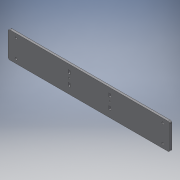
# Autodesk Inventor part: Motor Brace_1
Saved by Autodesk Inventor 2019 (Build 230136000, 136)
## iProperties
Created: 2020-03-11
Part Number: Motor Brace_1
Material: Generic
Document SubType Name: Modeling
Designer: Vijay
Density: 1 g/cm^3
Appearance: Default
Author: Vijay
Autodesk Inventor part; units mm, degrees
ref_plane "YZ Plane" through (0, 0, 0) normal (1, 0, 0) x (0, 1, 0)
ref_plane "XZ Plane" through (0, 0, 0) normal (0, 1, 0) x (-1, 0, 0)
ref_plane "XY Plane" through (0, 0, 0) normal (0, 0, 1) x (1, 0, 0)
sketch "Sketch1" plane through (0, 0, 0) normal (0, 0, 1) x (1, 0, 0)
  line L0 (-283, 0) -> (-283, -900) projected
  line L1 (26, 100) -> (26, -900) projected
  line L2 (-283, -450) -> (26, -450)
  line L3 (26, -450) -> (26, -400)
  line L4 (26, -400) -> (-283, -400)
  line L5 (-283, -400) -> (-283, -450)
  point P0 (0, 0)
  dimension "d0" = 50
  constraints: 8 end point, 2 midpoint, 2 parallel, 1 horizontal, 1 perpendicular
  measures "d0" distance between parallel lines of L2 L4
extrude "Extrusion1" add sketch "Sketch1" along normal blind 4
fillet "Fillet1" radius 3.175 4 edges at (-283, -450, 2) (-283, -400, 2) (26, -450, 2) (26, -400, 2)
sketch "Sketch2" plane through (0, 0, 4) normal (0, 0, 1) x (1, 0, 0)
  line L0 (-90.6012, -437.2508) -> (-90.6012, -431.2508) construction
  line L1 (-90.6012, -437.2508) -> (-86.6012, -437.2508) construction
  line L2 (-86.6012, -431.2508) -> (-86.6012, -437.2508) construction
  line L3 (-90.6012, -431.2508) -> (-86.6012, -431.2508) construction
  line L4 (-90.6012, -416.0508) -> (-90.6012, -410.0508) construction
  line L5 (-90.6012, -416.0508) -> (-86.6012, -416.0508) construction
  line L6 (-86.6012, -410.0508) -> (-86.6012, -416.0508) construction
  line L7 (-90.6012, -410.0508) -> (-86.6012, -410.0508) construction
  line L8 (-168.3754, -437.2508) -> (-168.3754, -431.2508) construction
  line L9 (-168.3754, -437.2508) -> (-164.3754, -437.2508) construction
  line L10 (-164.3754, -431.2508) -> (-164.3754, -437.2508) construction
  line L11 (-168.3754, -431.2508) -> (-164.3754, -431.2508) construction
  line L12 (-168.3754, -416.0508) -> (-168.3754, -410.0508) construction
  line L13 (-168.3754, -416.0508) -> (-164.3754, -416.0508) construction
  line L14 (-164.3754, -410.0508) -> (-164.3754, -416.0508) construction
  line L15 (-168.3754, -410.0508) -> (-164.3754, -410.0508) construction
  line L16 (-112.9543, -436.0142) -> (-107.1133, -436.0142) construction
  line L17 (-168.3754, -425.1508) -> (-168.3754, -422.1508) construction
  line L18 (-168.3754, -425.1508) -> (-168.3754, -422.1508) construction
  line L19 (-168.3754, -425.1508) -> (-164.3754, -425.1508) construction
  line L20 (-164.3754, -422.1508) -> (-164.3754, -425.1508) construction
  line L21 (-168.3754, -422.1508) -> (-164.3754, -422.1508) construction
  line L22 (-90.6012, -425.1508) -> (-90.6012, -422.1508) construction
  line L23 (-90.6012, -425.1508) -> (-86.6012, -425.1508) construction
  line L24 (-86.6012, -422.1508) -> (-86.6012, -425.1508) construction
  line L25 (-90.6012, -422.1508) -> (-86.6012, -422.1508) construction
  line L26 (-86.5012, -431.1508) -> (-86.5012, -437.3508)
  line L27 (-86.5012, -437.3508) -> (-90.7012, -437.3508)
  line L28 (-90.7012, -437.3508) -> (-90.7012, -431.1508)
  line L29 (-90.7012, -431.1508) -> (-86.5012, -431.1508)
  line L30 (-86.5012, -416.1508) -> (-90.7012, -416.1508)
  line L31 (-90.7012, -416.1508) -> (-90.7012, -409.9508)
  line L32 (-90.7012, -409.9508) -> (-86.5012, -409.9508)
  line L33 (-86.5012, -409.9508) -> (-86.5012, -416.1508)
  line L34 (-164.2754, -437.3508) -> (-168.4754, -437.3508)
  line L35 (-168.4754, -437.3508) -> (-168.4754, -431.1508)
  line L36 (-168.4754, -431.1508) -> (-164.2754, -431.1508)
  line L37 (-164.2754, -431.1508) -> (-164.2754, -437.3508)
  line L38 (-164.2754, -416.1508) -> (-168.4754, -416.1508)
  line L39 (-168.4754, -416.1508) -> (-168.4754, -409.9508)
  line L40 (-168.4754, -409.9508) -> (-164.2754, -409.9508)
  line L41 (-164.2754, -409.9508) -> (-164.2754, -416.1508)
  circle A0 centre (-166.3754, -423.6508) radius 1.5
  circle A1 centre (-88.6012, -423.6508) radius 1.5
  point P0 (0, 0)
  dimension "d4" = 0.1
  dimension "d5" = 0.1
  dimension "d6" = 0.1
  dimension "d7" = 0.1
  dimension "d8" = 3
  dimension "d9" = 3
  constraints: 32 end point, 2 centre point, 12 other
  measures "d4" distance between parallel lines of L3 L29
  measures "d5" distance between parallel lines of L5 L30
  measures "d6" distance between parallel lines of L9 L34
  measures "d7" distance between parallel lines of L13 L38
  measures "d8" diameter of A0
  measures "d9" diameter of A1
extrude "Extrusion2" cut sketch "Sketch2" against normal through all
sketch "Sketch3" plane through (0, 0, 4) normal (0, 0, 1) x (1, 0, 0)
  line L0 (17.1, 100) -> (17.1, -900) projected
  line L1 (8.9, 100) -> (17.1, 100) projected
  line L2 (8.9, 100) -> (8.9, -900) projected
  line L3 (17.1, -900) -> (8.9, -900) projected
  line L4 (-263.9, 100) -> (-263.9, -900) projected
  line L5 (-272.1, 100) -> (-263.9, 100) projected
  line L6 (-272.1, 100) -> (-272.1, -900) projected
  line L7 (-263.9, -900) -> (-272.1, -900) projected
  line L8 (55.4545, -442) -> (-299.148, -442) construction
  line L9 (72.1451, -408) -> (-299.148, -408) construction
  line L10 (-279.825, -450) -> (22.825, -450) construction
  line L11 (22.825, -400) -> (-279.825, -400) construction
  line L12 (13, -462.5908) -> (13, -387.796) construction
  line L13 (-268, -463.1777) -> (-268, -383.364) construction
  circle A0 centre (13, -442) radius 2
  circle A1 centre (13, -408) radius 2
  circle A2 centre (-268, -442) radius 2
  circle A3 centre (-268, -408) radius 2
  point P0 (0, 0)
  point P1 (-268, -900)
  point P2 (13, -900)
  dimension "d12" = 8
  dimension "d13" = 8
  dimension "d14" = 4
  dimension "d15" = 4
  dimension "d16" = 4
  dimension "d17" = 4
  constraints: 10 point on line, 8 end point, 4 centre point, 2 horizontal, 2 midpoint, 1 parallel, 1 vertical
  measures "d12" distance between parallel lines of L8 L10
  measures "d13" distance between parallel lines of L11 L9
  measures "d14" diameter of A0
  measures "d15" diameter of A1
  measures "d16" diameter of A2
  measures "d17" diameter of A3
extrude "Extrusion3" cut sketch "Sketch3" against normal blind 4 contours A0 | A1 | A2 | A3
body "Solid1"
